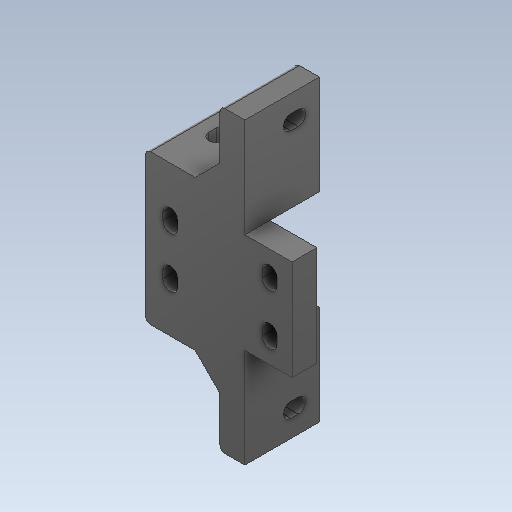
# Autodesk Inventor part: 0008-10-031 Suport L + placa
Saved by Autodesk Inventor 2020 (Build 240168000, 168)
## iProperties
Created: 2021-03-06
Part Number: 0008-10-031 Suport L + placa
Material: ABS Plastic
Document SubType Name: Modeling
Designer: Iulian Bors
Density: 1.06 g/cm^3
Appearance: Smooth - White
Mass: 68.8704 g
Surface Area: 185.276 cm^2
Volume: 64.972 cm^3
Description: Suport
Author: Iulian Bors
Subject: 031
Autodesk Inventor part; units mm, degrees
ref_plane "YZ Plane" through (0, 0, 0) normal (1, 0, 0) x (0, 1, 0)
ref_plane "XZ Plane" through (0, 0, 0) normal (0, 1, 0) x (-1, 0, 0)
sketch "Sketch1" plane through (0, 0, 0) normal (0, 0, 1) x (1, 0, 0)
  line L0 (-40, 5) -> (0, 5)
  line L1 (0, 5) -> (0, -5)
  line L2 (0, -5) -> (-40, -5)
  line L3 (-40, -5) -> (-40, 5)
  line L4 (-10, 35) -> (0, 35)
  line L5 (0, 35) -> (0, 5)
  line L6 (0, 5) -> (-10, 5)
  line L7 (-10, 5) -> (-10, 35)
  point P0 (0, 0)
  point P1 (0, 5)
  dimension "d0" = 10
  dimension "d1" = 40
  dimension "d2" = 40
  constraints: 16 end point, 4 parallel, 3 perpendicular, 2 horizontal, 1 collinear, 1 midpoint, 1 point on line
  measures "d0" distance of L2.end L0.start
  measures "d1" distance of L1.end L2.end
  measures "d2" distance between parallel lines of L2 L4
extrude "Extrusion1" add sketch "Sketch1" along normal blind 20
sketch "Sketch2" plane through (-10, 5, 0) normal (-1, 0, 0) x (0, 0, 1)
  line L0 (8.5, 20) -> (11.5, 20) construction
  line L1 (8.5, 17) -> (11.5, 17)
  line L2 (11.5, 23) -> (8.5, 23)
  arc A0 (8.5, 23) -> (8.5, 17) centre (8.5, 20) ccw
  arc A1 (11.5, 17) -> (11.5, 23) centre (11.5, 20) ccw
  line L3 (0, 30) -> (0, 0) projected
  line L4 (0, 30) -> (20, 30) projected
  line L5 (10, 21.547) -> (10, 15) construction
  line L6 (11.5, 20) -> (8.5, 20) construction
  line L7 (11.5, 17) -> (8.5, 17)
  line L8 (8.5, 23) -> (11.5, 23)
  arc A2 (11.5, 17) -> (11.5, 23) centre (11.5, 20) ccw
  arc A3 (8.5, 23) -> (8.5, 17) centre (8.5, 20) ccw
  point P0 (0, -5)
  point P1 (10, 20)
  point P2 (10, 18.2735)
  point P3 (10, 30)
  point P4 (10, 20)
  dimension "d5" = 6
  dimension "d6" = 3
  dimension "d7" = 10
  dimension "d8" = 10
  constraints: 18 end point, 8 point on circle, 7 symmetric about line, 4 centre point, 4 tangent, 3 midpoint, 1 horizontal, 1 parallel, 1 vertical, 1 vertical alignment, 2 other
  measures "d5" diameter of A1
  measures "d6" distance of L0.start L0.end
  measures "d7" distance from line of L3 point (10, 20)
  measures "d8" distance between parallel lines of L0 L4
extrude "Extrusion2" cut sketch "Sketch2" against normal through all
sketch "Sketch3" plane through (-40, 5, 0) normal (0, 1, 0) x (1, 0, 0)
  line L0 (10, -8.5) -> (10, -11.5) construction
  line L1 (7, -8.5) -> (7, -11.5)
  line L2 (13, -11.5) -> (13, -8.5)
  arc A0 (13, -8.5) -> (7, -8.5) centre (10, -8.5) ccw
  arc A1 (7, -11.5) -> (13, -11.5) centre (10, -11.5) ccw
  line L3 (30, 0) -> (0, 0) projected
  line L4 (0, 0) -> (0, -20) projected
  line L5 (15.2557, -10) -> (9.287, -10) construction
  line L6 (10, -11.5) -> (10, -8.5) construction
  line L7 (7, -11.5) -> (7, -8.5)
  line L8 (13, -8.5) -> (13, -11.5)
  arc A2 (7, -11.5) -> (13, -11.5) centre (10, -11.5) ccw
  arc A3 (13, -8.5) -> (7, -8.5) centre (10, -8.5) ccw
  point P0 (40, 0)
  point P1 (10, -10)
  point P2 (12.2713, -10)
  point P3 (0, -10)
  point P4 (10, -10)
  dimension "d11" = 3
  dimension "d12" = 6
  dimension "d13" = 10
  dimension "d14" = 10
  constraints: 18 end point, 8 point on circle, 7 symmetric about line, 4 centre point, 4 tangent, 3 midpoint, 1 horizontal, 1 horizontal alignment, 1 parallel, 1 vertical, 2 other
  measures "d11" distance of L0.start L0.end
  measures "d12" distance between parallel lines of L1 L2
  measures "d13" distance from line of L3 point (10, -10)
  measures "d14" distance between parallel lines of L4 L0
extrude "Extrusion3" cut sketch "Sketch3" against normal through all
chamfer "Chamfer1" distance 10 angle 45 1 edges at (-10, 5, 10)
sketch "Sketch10" plane through (0, 0, 20) normal (0, 0, 1) x (1, 0, 0)
  line L0 (-40, -85.3) -> (0, -85.3)
  line L1 (0, -85.3) -> (0, 35)
  line L2 (0, 35) -> (-40, 35)
  line L3 (-40, 35) -> (-40, -85.3)
  line L4 (-40, 5) -> (-40, -5) projected
  line L5 (0, 35) -> (-10, 35) projected
  line L6 (0, -5) -> (0, 35) projected
  line L7 (-40, -5) -> (0, -5) projected
  line L8 (0, -45.3) -> (19, -45.3)
  line L9 (19, -45.3) -> (19, -5)
  line L10 (19, -5) -> (0, -5)
  line L11 (0, -5) -> (0, -45.3)
  point P0 (0, 0)
  dimension "d30" = 80.3
  dimension "d31" = 120.3
  dimension "d37" = 40.3
  dimension "d38" = 19
  constraints: 16 end point, 5 collinear, 4 parallel, 2 horizontal, 2 perpendicular
  measures "d30" distance between parallel lines of L7 L0
  measures "d31" distance of L2.end L0.start
  measures "d37" distance of L8.end L9.end
  measures "d38" distance between parallel lines of L9 L1
extrude "Extrusion7" add sketch "Sketch10" along normal blind 10
ref_plane "Work Plane2" through (-10, -25.15, 0) normal (0, 1, 0) x (1, 0, 0)
mirror "Mirror2" about plane through (-10, -25.15, 0) normal (0, 1, 0) of "Extrusion1", "Extrusion2", "Extrusion3", "Chamfer1"
sketch "Sketch11" plane through (0, 0, 20) normal (0, 0, -1) x (-1, 0, 0)
  line L0 (10, 35) -> (10, 15) projected
  line L1 (20, 5) -> (10, 15) projected
  line L2 (20, 5) -> (40, 5) projected
  line L3 (40, 35) -> (40, 5) projected
  line L4 (10, 35) -> (40, 35) projected
  point P0 (0, 0)
extrude "Extrusion8" cut sketch "Sketch11" against normal through all
mirror "Mirror3" about plane through (-10, -25.15, 0) normal (0, 1, 0) of "Extrusion8"
sketch "Sketch12" plane through (0, 0, 20) normal (0, 0, -1) x (-1, 0, 0)
  line L0 (30, -13.5) -> (30, -16.5) construction
  line L1 (27, -13.5) -> (27, -16.5)
  line L2 (33, -16.5) -> (33, -13.5)
  arc A0 (33, -13.5) -> (27, -13.5) centre (30, -13.5) ccw
  arc A1 (27, -16.5) -> (33, -16.5) centre (30, -16.5) ccw
  line L3 (40, -5) -> (40, -45.3) projected
  line L4 (40, -5) -> (0, -5) projected
  line L5 (-10, -13.5) -> (-10, -16.5) construction
  line L6 (-13, -13.5) -> (-13, -16.5)
  line L7 (-7, -16.5) -> (-7, -13.5)
  arc A2 (-7, -13.5) -> (-13, -13.5) centre (-10, -13.5) ccw
  arc A3 (-13, -16.5) -> (-7, -16.5) centre (-10, -16.5) ccw
  line L8 (-19, -45.3) -> (-19, -5) projected
  line L9 (33, -25.15) -> (24.6871, -25.15) construction
  line L10 (30, -36.8) -> (30, -33.8) construction
  line L11 (27, -36.8) -> (27, -33.8)
  line L12 (33, -33.8) -> (33, -36.8)
  arc A4 (27, -36.8) -> (33, -36.8) centre (30, -36.8) ccw
  arc A5 (33, -33.8) -> (27, -33.8) centre (30, -33.8) ccw
  line L13 (-10, -36.8) -> (-10, -33.8) construction
  line L14 (-13, -36.8) -> (-13, -33.8)
  line L15 (-7, -33.8) -> (-7, -36.8)
  arc A6 (-13, -36.8) -> (-7, -36.8) centre (-10, -36.8) ccw
  arc A7 (-7, -33.8) -> (-13, -33.8) centre (-10, -33.8) ccw
  point P0 (0, 0)
  point P1 (30, -15)
  point P2 (-10, -15)
  point P3 (28.8435, -25.15)
  point P4 (40, -25.15)
  point P5 (30, -35.3)
  point P6 (-10, -35.3)
  dimension "d39" = 3
  dimension "d40" = 10
  dimension "d41" = 10
  dimension "d42" = 6
  dimension "d43" = 9
  constraints: 34 end point, 16 point on circle, 14 symmetric about line, 8 centre point, 8 tangent, 4 midpoint, 3 parallel, 2 horizontal alignment, 2 vertical, 1 equal radius, 1 horizontal, 4 other
  measures "d39" distance of L0.start L0.end
  measures "d40" distance from line of point (30, -15) L3
  measures "d41" distance from line of L4 point (30, -15)
  measures "d42" distance between parallel lines of L1 L2
  measures "d43" distance from line of L8 L5.end
extrude "Extrusion9" cut sketch "Sketch12" against normal through all
fillet "Fillet2" radius 2 3 edges at (-40, 5, 15) (-10, 35, 15) (-10, -85.3, 15)
equation "\"d2\" = d1"
body "Solid1"
